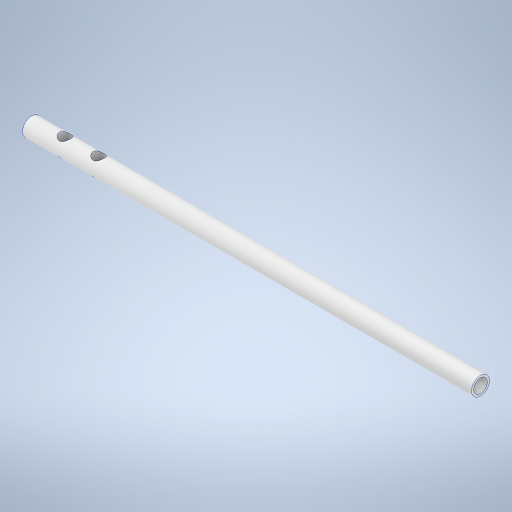
# Autodesk Inventor part: counterweight-rod
Saved by Autodesk Inventor 2024 (Build 280153000, 153)
## iProperties
Created: 2025-12-27
Part Number: counterweight-rod
Material: Aluminum 6061
Document SubType Name: Modeling
Designer: schar
Density: 2.7 g/cm^3
Appearance: Aluminum - Flat
Author: schar
Autodesk Inventor part; units mm, degrees
ref_plane "YZ Plane" through (0, 0, 0) normal (1, 0, 0) x (0, 1, 0)
ref_plane "XY Plane" through (0, 0, 0) normal (0, 0, 1) x (1, 0, 0)
sketch "Sketch1" plane through (0, 0, 0) normal (1, 0, 0) x (0, 1, 0)
  circle A0 centre (0, 0) radius 4
  dimension "d0" = 8
  constraints: 1 centre point, 1 coincident
  measures "d0" diameter of A0
extrude "Extrusion1" add sketch "Sketch1" along normal blind 200
sketch "Sketch2" plane through (0, 0, 0) normal (0, 1, 0) x (-1, 0, 0)
  line L0 (0, 0) -> (-15, 0)
  line L1 (-15, 0) -> (-30, 0)
  circle A0 centre (-30, 0) radius 2.5
  circle A1 centre (-15, 0) radius 2.5
  dimension "d3" = 15
  dimension "d4" = 15
  dimension "d5" = 5
  dimension "d6" = 5
  constraints: 4 end point, 2 centre point, 2 coincident, 1 horizontal, 1 point on line
  measures "d3" distance of L0.start L0.end
  measures "d4" distance of L0.end L1.end
  measures "d5" diameter of A0
  measures "d6" diameter of A1
extrude "Extrusion2" cut sketch "Sketch2" along normal mid plane 200
sketch "Sketch3" plane through (200, 0, 0) normal (1, 0, 0) x (0, 0, -1)
  circle A0 centre (0, 0) radius 3
  dimension "d9" = 6
  constraints: 1 centre point, 1 coincident
  measures "d9" diameter of A0
extrude "Extrusion3" cut sketch "Sketch3" against normal blind 20
thread "Thread1" size "M6x1" class "6H" standard "ANSI Metric M Profile" length 15
ref_plane "Work Plane2" through (0, -4, 0) normal (0, 1, 0) x (-1, 0, 0)
sketch "Sketch4" plane through (0, -4, 0) normal (0, 1, 0) x (-1, 0, 0)
  line L0 (0, 4) -> (0, -4) projected
  line L1 (0, -4) -> (-200, -4) projected
  line L2 (0, 4) -> (-40, 4)
  line L3 (-40, 4) -> (-40, -4)
  line L4 (-40, -4) -> (0, -4)
  line L5 (0, -4) -> (0, 4)
  point P0 (0, 0)
  dimension "d16" = 40
  constraints: 8 end point, 2 parallel, 1 horizontal, 1 perpendicular, 1 point on line
  measures "d16" distance of L4.end L3.end
extrude "Extrusion4" cut sketch "Sketch4" along normal blind 0.5
body "Solid1"
